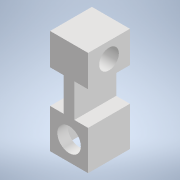
# Autodesk Inventor part: shuttle
Saved by Autodesk Inventor 2020 (Build 240168000, 168)
## iProperties
Created: 2019-11-08
Part Number: shuttle
Material: Generic
Document SubType Name: Modeling
Designer: Hymowitz
Density: 1 g/cm^3
Appearance: Default
Author: Hymowitz
Autodesk Inventor part; units mm, degrees
ref_plane "YZ Plane" through (0, 0, 0) normal (1, 0, 0) x (0, 1, 0)
ref_plane "XZ Plane" through (0, 0, 0) normal (0, 1, 0) x (-1, 0, 0)
ref_plane "XY Plane" through (0, 0, 0) normal (0, 0, 1) x (1, 0, 0)
sketch "Sketch2" plane through (0, 0, 0) normal (0, 0, 1) x (1, 0, 0)
  line L0 (1, 3.175) -> (1, -18.8331) construction
  line L1 (1.8, -9.8341) -> (0.2, -9.8341)
  line L2 (1.8, -3.8841) -> (1.8, 5.975) construction
  line L3 (1.8, 5.975) -> (3.8868, 5.975)
  line L4 (3.8868, 5.975) -> (3.8868, 1.2)
  line L5 (3.8868, 1.2) -> (1.8, 1.2)
  line L6 (0.2, 1.2) -> (-1.8868, 1.2)
  line L7 (-1.8868, 1.2) -> (-1.8868, 5.975)
  line L8 (-1.8868, 5.975) -> (1.8, 5.975)
  line L9 (-1.8868, -3.8841) -> (-1.8868, -9.8341)
  line L10 (-1.8868, -9.8341) -> (3.8868, -9.8341)
  line L11 (3.8868, -9.8341) -> (3.8868, -3.8841)
  line L12 (3.8868, -3.8841) -> (-1.8868, -9.8341) construction
  line L13 (-1.8868, -3.8841) -> (3.8868, -9.8341) construction
  line L14 (1.8, 1.2) -> (1.8, -3.8841)
  line L15 (0.2, -3.8841) -> (0.2, 1.2)
  line L16 (3.8868, -3.8841) -> (1.8, -3.8841)
  line L17 (0.2, -3.8841) -> (-1.8868, -3.8841)
  line L18 (4.175, 6.175) -> (4.175, 1) construction
  line L19 (4.175, 6.175) -> (-2.939, 6.175) construction
  line L20 (4.175, 1) -> (-2.939, 1) construction
  line L21 (4.175, -3.6841) -> (4.175, -10.0341) construction
  line L22 (4.175, -3.6841) -> (5.7142, -3.6841) construction
  line L23 (4.175, -10.0341) -> (5.7142, -10.0341) construction
  line L24 (2, 1) -> (2, -3.6841) construction
  line L25 (0, 1) -> (0, -3.6841) construction
  point P0 (1, -6.8591)
  point P1 (0.2, -9.8341)
  point P2 (1.8, -9.8341)
  dimension "d15" = 0.2
  dimension "d16" = 0.2
  dimension "d17" = 0.2
  dimension "d18" = 0.2
  dimension "d19" = 0.2
  dimension "d20" = 0.2
  constraints: 44 end point, 9 horizontal, 7 perpendicular, 4 collinear, 4 parallel, 4 point on line, 2 midpoint, 1 coincident, 1 vertical, 2 other
  measures "d15" distance between parallel lines of L8 L19
  measures "d16" distance between parallel lines of L20 L6
  measures "d17" distance between parallel lines of L23 L10
  measures "d18" distance between parallel lines of L16 L22
  measures "d19" distance between parallel lines of L25 L15
  measures "d20" distance between parallel lines of L24 L2
extrude "Extrusion1" add sketch "Sketch2" along normal blind 6.35
sketch "Sketch3" plane through (0, 0, 6.35) normal (0, 0, 1) x (1, 0, 0)
  circle A0 centre (1, -6.8591) radius 1.5875 construction
  circle A1 centre (1, -6.8591) radius 1.7875
  point P0 (0, 0)
  dimension "d9" = 0.2
  constraints: 2 centre point, 2 other
  measures "d9" radial gap between concentric circles of A0 A1
extrude "Extrusion2" cut sketch "Sketch3" against normal through all
sketch "Sketch4" plane through (3.8868, 1.2, 0) normal (1, 0, 0) x (0, 0, -1)
  line L0 (-6.35, 0) -> (-6.35, 4.775) construction
  line L1 (-6.35, 2.3875) -> (0, 2.3875) construction
  circle A0 centre (-3.175, 2.3875) radius 1.5
  point P0 (0, -1.2)
  dimension "d12" = 3
  constraints: 2 end point, 2 midpoint, 1 centre point, 1 horizontal
  measures "d12" diameter of A0
extrude "Extrusion3" cut sketch "Sketch4" against normal through all
sketch "Sketch5" plane through (-1.8868, -9.8341, 0) normal (0, -1, 0) x (1, 0, 0)
  line L0 (0, 0) -> (0, 6.35) construction
  line L1 (3.6868, 0) -> (5.7737, 0) construction
  line L2 (0, 6.35) -> (5.7737, 0) construction
  line L3 (0.24, 1.5797) -> (5.5337, 1.5797)
  line L4 (5.5337, 1.5797) -> (5.5337, 4.7703)
  line L5 (5.5337, 4.7703) -> (0.24, 4.7703)
  line L6 (0.24, 4.7703) -> (0.24, 1.5797)
  line L7 (0.24, 1.5797) -> (5.5337, 4.7703) construction
  line L8 (5.5337, 1.5797) -> (0.24, 4.7703) construction
  point P0 (1.8868, 0)
  point P1 (2.8868, 3.175)
  dimension "d21" = 5.2937
  dimension "d22" = 3.1907
  constraints: 14 end point, 3 midpoint, 2 parallel, 1 horizontal, 1 perpendicular
  measures "d21" distance of L4.end L5.end
  measures "d22" distance of L3.end L4.end
extrude "Extrusion4" cut sketch "Sketch5" against normal blind 4.15
body "Solid1"
